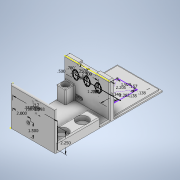
# Autodesk Inventor part: electropneumatic tray - rev2
Saved by Autodesk Inventor 2020 (Build 240168000, 168)
## iProperties
Created: 2022-01-12
Part Number: electropneumatic tray - rev2
Material: Generic
Document SubType Name: Modeling
Designer: pab2
Density: 1 g/cm^3
Appearance: Default
Author: pab2
Autodesk Inventor part; units mm, degrees
ref_plane "YZ Plane" through (0, 0, 0) normal (1, 0, 0) x (0, 1, 0)
ref_plane "XZ Plane" through (0, 0, 0) normal (0, 1, 0) x (-1, 0, 0)
ref_plane "XY Plane" through (0, 0, 0) normal (0, 0, 1) x (1, 0, 0)
sketch "Sketch1" plane through (0, 0, 0) normal (0, 0, 1) x (1, 0, 0)
  line L0 (0, 0) -> (127, 0)
  line L1 (127, 0) -> (127, 101.6)
  line L2 (127, 101.6) -> (0, 101.6)
  line L3 (0, 101.6) -> (0, 0)
  dimension "d0" = 127
  dimension "d1" = 101.6
  constraints: 8 end point, 2 parallel, 1 horizontal, 1 perpendicular
  measures "d0" distance of L2.end L1.end
  measures "d1" distance of L1.end L0.end
extrude "Extrusion1" add sketch "Sketch1" along normal blind 12.7
sketch "Sketch2" plane through (0, 0, 12.7) normal (0, 0, 1) x (1, 0, 0)
  line L0 (127, 101.6) -> (0, 101.6) projected
  line L1 (63.5, 101.6) -> (63.5, 69.85)
  line L2 (63.5, 69.85) -> (95.25, 69.85)
  line L3 (95.25, 69.85) -> (31.75, 69.85)
  circle A0 centre (31.75, 69.85) radius 9.906
  circle A1 centre (95.25, 69.85) radius 9.906
  line L4 (31.75, 63.5) -> (31.75, 76.2) construction
  line L5 (38.1, 63.5) -> (38.1, 76.2)
  line L6 (25.4, 76.2) -> (25.4, 63.5)
  arc A2 (25.4, 63.5) -> (38.1, 63.5) centre (31.75, 63.5) ccw
  arc A3 (38.1, 76.2) -> (25.4, 76.2) centre (31.75, 76.2) ccw
  line L7 (127, 69.85) -> (63.5, 69.85)
  circle A4 centre (63.5, 69.85) radius 9.906
  line L8 (69.85, 63.5) -> (69.85, 76.2)
  line L9 (57.15, 76.2) -> (57.15, 63.5)
  arc A5 (69.85, 76.2) -> (57.15, 76.2) centre (63.5, 76.2) ccw
  arc A6 (57.15, 63.5) -> (69.85, 63.5) centre (63.5, 63.5) ccw
  line L10 (158.75, 69.85) -> (95.25, 69.85)
  circle A7 centre (95.25, 69.85) radius 9.906
  line L11 (101.6, 63.5) -> (101.6, 76.2)
  line L12 (88.9, 76.2) -> (88.9, 63.5)
  arc A8 (101.6, 76.2) -> (88.9, 76.2) centre (95.25, 76.2) ccw
  arc A9 (88.9, 63.5) -> (101.6, 63.5) centre (95.25, 63.5) ccw
  point P0 (0, 0)
  point P1 (57.301, 62.1233)
  point P2 (69.699, 62.1233)
  point P3 (69.699, 77.5767)
  point P4 (57.301, 77.5767)
  dimension "d4" = 31.75
  dimension "d5" = 31.75
  dimension "d6" = 63.5
  dimension "d7" = 19.812
  dimension "d9" = 19.812
  dimension "d12" = 6.35
  dimension "d13" = 12.7
  dimension "d16" = 31.75
  constraints: 26 end point, 12 point on circle, 10 centre point, 4 coincident, 4 tangent, 2 midpoint, 2 perpendicular, 1 collinear, 1 horizontal, 1 parallel, 1 point on line, 1 vertical, 29 other
  measures "d4" distance of L1.start L1.end
  measures "d5" distance of L1.end L2.end
  measures "d6" distance of L2.end L3.end
  measures "d7" diameter of A0
  measures "d9" diameter of A1
  measures "d12" distance of A0.centre L4.end
  measures "d13" diameter of A3
  measures "d16" distance of L3.end L7.end
sketch "Sketch3" plane through (0, 0, 12.7) normal (0, 0, 1) x (1, 0, 0)
  line L0 (0, 101.6) -> (0, 0) projected
  line L1 (0, 0) -> (127, 0)
  line L2 (127, 0) -> (127, 6.35)
  line L3 (127, 6.35) -> (0, 6.35)
  line L4 (0, 6.35) -> (0, 0)
  dimension "d23" = 127
  dimension "d24" = 6.35
  constraints: 8 end point, 2 parallel, 1 horizontal, 1 perpendicular
  measures "d23" distance of L3.end L2.end
  measures "d24" distance of L2.end L1.end
extrude "Extrusion4" add sketch "Sketch3" along normal blind 152.4
sketch "Sketch4" plane through (0, 6.35, 12.7) normal (0, 1, 0) x (1, 0, 0)
  line L0 (127, 12.7) -> (127, -152.4) projected
  line L1 (0, 0) -> (0, -152.4) projected
  line L2 (127, -152.4) -> (0, -152.4)
  line L3 (0, -152.4) -> (0, -146.05)
  line L4 (0, -146.05) -> (127, -146.05)
  line L5 (127, -146.05) -> (127, -152.4)
  point P0 (0, 12.7)
  point P1 (0, -152.4)
  dimension "d27" = 6.35
  constraints: 8 end point, 2 parallel, 1 horizontal, 1 perpendicular, 1 point on line
  measures "d27" distance of L2.end L3.end
extrude "Extrusion5" add sketch "Sketch4" along normal blind 101.6
sketch "Sketch5" plane through (127, 6.35, 158.75) normal (0, 0, -1) x (-1, 0, 0)
  line L0 (127, 0) -> (127, 101.6) projected
  line L1 (127, 0) -> (0, 0)
  line L2 (0, 0) -> (0, 57.15)
  line L3 (0, 57.15) -> (127, 57.15)
  line L4 (127, 57.15) -> (127, 0)
  line L5 (63.5, 57.15) -> (63.5, 89.9922)
  line L6 (63.5, 57.15) -> (96.3422, 57.15) construction
  line L7 (63.5, 57.15) -> (72.5424, 57.15)
  line L8 (72.5424, 57.15) -> (72.5424, 65.6082)
  line L9 (72.5424, 65.6082) -> (54.4576, 65.6082)
  line L10 (127, 95.25) -> (127, -6.35) projected
  line L11 (127, -6.35) -> (76.2, -6.35)
  line L12 (76.2, -6.35) -> (76.2, 31.75)
  line L13 (76.2, 31.75) -> (127, 31.75)
  line L14 (127, 31.75) -> (127, -6.35)
  dimension "d30" = 127
  dimension "d31" = 57.15
  dimension "d32" = 32.8422
  dimension "d33" = 90
  dimension "d34" = 9.0424
  dimension "d35" = 8.4582
  dimension "d36" = 18.0848
  dimension "d120" = 50.8
  dimension "d121" = 38.1
  constraints: 26 end point, 5 perpendicular, 4 parallel, 3 horizontal, 1 coincident, 1 midpoint, 1 point on line, 1 vertical
  measures "d30" distance of L2.end L3.end
  measures "d31" distance of L1.end L2.end
  measures "d32" distance of L5.start L5.end
  measures "d33" angle of L6 L5
  measures "d34" distance of L5.start L7.end
  measures "d35" distance of L7.end L8.end
  measures "d36" distance of L8.end L9.end
  measures "d120" distance of L12.end L13.end
  measures "d121" distance of L11.end L12.end
hole "Hole1" at (63.5, 96.3422, 158.75) at (54.4576, 71.9582, 158.75) at (72.5424, 71.9582, 158.75) direction (0, 0, 1) diameter 3.4036 end through all clearance for "Socket Head Cap Screw" size "M3" standard "Ansi Metric M Profile"
sketch "Sketch10" plane through (0, 6.35, 12.7) normal (0, 1, 0) x (1, 0, 0)
  line L0 (127, 0) -> (127, -25.4)
  line L1 (127, 12.7) -> (127, -152.4) projected
  line L2 (127, -25.4) -> (88.9, -25.4)
  line L3 (88.9, -25.4) -> (88.9, -152.4)
  line L4 (88.9, -152.4) -> (127, -152.4)
  line L5 (127, -152.4) -> (127, -25.4)
  point P0 (0, 12.7)
  dimension "d58" = 25.4
  dimension "d59" = 38.1
  dimension "d60" = 127
  constraints: 10 end point, 2 parallel, 1 horizontal, 1 perpendicular, 1 point on line
  measures "d58" distance of L0.start L0.end
  measures "d59" distance of L4.end L3.end
  measures "d60" distance of L3.end L2.end
extrude "Extrusion9" add sketch "Sketch10" along normal blind 19.05
sketch "Sketch11" plane through (0, 25.4, 12.7) normal (0, 1, 0) x (1, 0, 0)
  line L0 (127, -25.4) -> (88.9, -25.4) projected
  line L1 (107.95, -25.4) -> (120.65, -25.4) construction
  circle A0 centre (107.95, -114.3) radius 16.51
  circle A1 centre (107.95, -57.15) radius 16.51
  line L2 (107.95, -25.4) -> (107.95, -57.15)
  line L3 (107.95, -25.4) -> (139.7, -25.4) construction
  line L4 (127, -146.05) -> (0, -146.05) projected
  line L5 (107.95, -146.05) -> (107.95, -114.3)
  line L6 (107.95, -146.05) -> (139.7, -146.05) construction
  point P0 (0, 12.7)
  dimension "d69" = 33.02
  dimension "d70" = 33.02
  dimension "d115" = 31.75
  dimension "d116" = 90
  dimension "d117" = 31.75
  dimension "d118" = 90
  constraints: 10 end point, 3 horizontal, 3 perpendicular, 2 centre point, 2 coincident, 1 midpoint, 1 point on line, 1 vertical
  measures "d69" diameter of A0
  measures "d70" diameter of A1
  measures "d115" distance of L1.start L2.end
  measures "d116" angle of L2 L3
  measures "d117" distance of L5.start L5.end
  measures "d118" angle of L6 L5
extrude "Extrusion10" cut sketch "Sketch11" against normal blind 12.7
sketch "Sketch12" plane through (0, 0, 0) normal (0, 0, -1) x (-1, 0, 0)
  line L0 (-127, 6.35) -> (-88.9, 6.35) projected
  line L1 (-127, 6.35) -> (0, 6.35)
  line L2 (0, 6.35) -> (0, 0)
  line L3 (0, 0) -> (-127, 0)
  line L4 (-127, 0) -> (-127, 6.35)
  constraints: 8 end point, 2 parallel, 1 horizontal, 1 perpendicular
extrude "Extrusion11" add sketch "Sketch12" along normal blind 137.16
sketch "Sketch13" plane through (0, 6.35, 0) normal (0, 1, 0) x (1, 0, 0)
  line L0 (35.5, 16.5925) -> (35.5, 101.5925)
  line L1 (35.5, 101.5925) -> (91.5, 101.5925)
  line L2 (91.5, 101.5925) -> (91.5, 16.5925)
  line L3 (91.5, 16.5925) -> (35.5, 16.5925)
  line L4 (35.5, 16.5925) -> (91.5, 101.5925) construction
  line L5 (35.5, 101.5925) -> (91.5, 16.5925) construction
  line L6 (91.5, 101.5925) -> (91.5, 98.0925)
  line L7 (91.5, 98.0925) -> (88, 98.0925)
  line L8 (88, 98.0925) -> (88, 101.5925)
  line L9 (88, 101.5925) -> (91.5, 101.5925)
  circle A0 centre (88, 98.0925) radius 2
  circle A1 centre (39, 98.0925) radius 2
  circle A2 centre (88, 40.0925) radius 2
  circle A3 centre (39, 40.0925) radius 2
  point P0 (0, 0)
  point P1 (63.5, 59.0925)
  dimension "d75" = 85
  dimension "d76" = 56
  dimension "d77" = 3.5
  dimension "d78" = 3.5
  dimension "d79" = 4
  dimension "d82" = 49
  dimension "d85" = 58
  constraints: 20 end point, 4 centre point, 4 coincident, 4 parallel, 2 midpoint, 2 perpendicular, 1 horizontal, 1 vertical, 9 other
  measures "d75" distance of L1.end L2.end
  measures "d76" distance of L0.end L1.end
  measures "d77" distance of L7.end L8.end
  measures "d78" distance of L6.end L7.end
  measures "d79" diameter of A0
  measures "d82" distance of A0.centre A1.centre
  measures "d85" distance of A0.centre A2.centre
extrude "Extrusion12" add sketch "Sketch13" along normal blind 3.175 contours A0 L7 L8 | L8 L7 A0 | A1 | A2 | A3
hole "Hole2" at (88, 6.35, -98.0925) at (39, 6.35, -98.0925) at (88, 6.35, -40.0925) at (39, 6.35, -40.0925) direction (0, 1, 0) diameter 2.013 depth 7.5946 tip angle 118 thread size "M2.5x0.45" class "6H" standard "ANSI Metric M Profile"
sketch "Sketch14" plane through (0, 6.35, 0) normal (0, 1, 0) x (1, 0, 0)
  line L0 (0, 137.16) -> (127, 137.16) projected
  line L1 (0, 0) -> (5.08, 0)
  line L2 (5.08, 0) -> (5.08, 137.16)
  line L3 (5.08, 137.16) -> (0, 137.16)
  line L4 (0, 137.16) -> (0, 0)
  line L5 (0, 137.16) -> (0, -165.1) projected
  line L6 (0, 137.16) -> (127, 137.16)
  line L7 (127, 137.16) -> (127, 132.08)
  line L8 (127, 132.08) -> (0, 132.08)
  line L9 (0, 132.08) -> (0, 137.16)
  line L10 (127, 137.16) -> (127, -165.1) projected
  line L11 (127, 0) -> (0, 0) projected
  line L12 (127, 137.16) -> (121.92, 137.16)
  line L13 (121.92, 137.16) -> (121.92, 0)
  line L14 (121.92, 0) -> (127, 0)
  line L15 (127, 0) -> (127, 137.16)
  point P0 (5.08, 132.08)
  point P1 (121.92, 132.08)
  dimension "d97" = 5.08
  dimension "d98" = 127
  dimension "d99" = 5.08
  dimension "d100" = 5.08
  constraints: 24 end point, 6 parallel, 3 horizontal, 3 perpendicular, 2 point on line
  measures "d97" distance of L3.end L2.end
  measures "d98" distance of L7.end L8.end
  measures "d99" distance of L6.end L7.end
  measures "d100" distance of L14.end L13.end
extrude "Extrusion13" cut sketch "Sketch14" against normal blind 3.175 contours L0 L2 L8 L4 | L0 L13 L8 L2 | L8 L2 L1 L4 | L0 L7 L8 L13 | L8 L10 L11 L13
sketch "Sketch15" plane through (0, 101.6, 0) normal (0, 1, 0) x (1, 0, 0)
  line L0 (121.92, 0) -> (5.08, 0) projected
  line L1 (63.5, 0) -> (63.5, -7.62)
  line L2 (88.9, -15.24) -> (38.1, -15.24)
  line L3 (38.1, -15.24) -> (38.1, 0)
  line L4 (38.1, 0) -> (88.9, 0)
  line L5 (88.9, 0) -> (88.9, -15.24)
  line L6 (88.9, -15.24) -> (38.1, 0) construction
  line L7 (38.1, -15.24) -> (88.9, 0) construction
  point P0 (0, 0)
  dimension "d103" = 7.62
  dimension "d104" = 50.8
  constraints: 14 end point, 3 midpoint, 2 parallel, 1 horizontal, 1 perpendicular, 1 point on line, 1 vertical
  measures "d103" distance of L1.start L1.end
  measures "d104" distance of L3.end L4.end
extrude "Extrusion14" cut sketch "Sketch15" against normal blind 5.08
sketch "Sketch16" plane through (0, 96.52, 0) normal (0, 1, 0) x (1, 0, 0)
  line L0 (38.1, -12.7) -> (38.1, 0) projected
  line L1 (38.1, 0) -> (63.5, 0)
  line L2 (121.92, 0) -> (5.08, 0) projected
  line L3 (63.5, 0) -> (63.5, -7.62)
  point P0 (0, 0)
  point P1 (38.1, -15.24)
  constraints: 4 end point, 1 midpoint, 1 vertical
hole "Hole3" at (63.5, 96.52, 7.62) direction (0, -1, 0) diameter 4.9784 depth 6.35 tip angle 118 thread size "1/4-20 UNC" class "2B" standard "ANSI Unified Screw Threads"
fillet "Fillet1" radius 3.175 11 edges at (0, 101.6, 6.35) (107.95, 101.6, 12.7) (19.05, 101.6, 12.7) (127, 101.6, 6.35) (127, 53.975, 12.7) (127, 6.35, 25.4) (0, 6.35, 85.725) (127, 66.675, 158.75) (63.5, 107.95, 158.75) (0, 57.15, 158.75) (63.5, 107.95, 165.1)
fillet "Fillet2" radius 3.175 7 edges at (127, 4.7628, 38.1) (127, 15.875, 38.1) (107.95, 25.4, 38.1) (127, 25.4, 98.425) (127, 25.4, 160.3372) (88.9, 25.4, 98.425) (88.9, 15.875, 38.1)
sketch "Sketch17" plane through (0, 0, 165.1) normal (0, 0, 1) x (1, 0, 0)
  point P0 (0, 0)
sketch "Sketch18" plane through (3.175, 6.35, 12.7) normal (0, 1, 0) x (1, 0, 0)
  line L0 (0, -146.05) -> (0, 0) projected
  line L1 (0, 0) -> (25.4, 0)
  line L2 (25.4, 0) -> (25.4, -25.4)
  line L3 (25.4, -25.4) -> (0, -25.4)
  line L4 (0, -25.4) -> (0, 0)
  point P0 (-3.175, 12.7)
  dimension "d129" = 25.4
  dimension "d130" = 25.4
  constraints: 8 end point, 2 parallel, 1 horizontal, 1 perpendicular
  measures "d129" distance of L2.end L3.end
  measures "d130" distance of L1.end L2.end
extrude "Extrusion15" add sketch "Sketch18" along normal blind 38.1
hole "Hole4" at (50.8, 38.1, 158.75) direction (0, 0, 1) diameter 8.89 end through all
sketch "Sketch19" plane through (3.175, 44.45, 12.7) normal (0, 1, 0) x (1, 0, 0)
  line L0 (25.4, -25.4) -> (0, -25.4) projected
  line L1 (0, -25.4) -> (12.7, -25.4)
  line L2 (12.7, -25.4) -> (12.7, -12.7)
  circle A0 centre (12.7, -12.7) radius 9.906
  point P0 (-3.175, 12.7)
  dimension "d133" = 12.7
  dimension "d134" = 12.7
  dimension "d135" = 90
  dimension "d136" = 19.812
  constraints: 4 end point, 1 centre point, 1 coincident, 1 midpoint, 1 perpendicular
  measures "d133" distance of L0.end L1.end
  measures "d134" distance of L1.end L2.end
  measures "d135" angle of L2 L1
  measures "d136" diameter of A0
extrude "Extrusion16" cut sketch "Sketch19" against normal blind 25.4
sketch "Sketch20" plane through (0, 0, 0) normal (0, 0, -1) x (-1, 0, 0)
  line L0 (-3.175, 44.45) -> (-28.575, 44.45) projected
  line L1 (-28.575, 44.45) -> (-28.575, 6.35) projected
  line L2 (-3.175, 6.35) -> (-3.175, 44.45) projected
  line L3 (-3.175, 6.35) -> (-3.175, 44.45) projected
  line L4 (-3.175, 44.45) -> (-28.575, 44.45) projected
  line L5 (-15.875, 44.45) -> (-15.875, 19.05)
  line L6 (-25.781, 19.05) -> (-5.969, 19.05) projected
  circle A0 centre (-15.875, 19.05) radius 3.175
  line L7 (-15.875, 19.05) -> (-41.275, 19.05)
  line L8 (-47.625, 19.05) -> (-34.925, 19.05) construction
  line L9 (-47.625, 15.875) -> (-34.925, 15.875)
  line L10 (-34.925, 22.225) -> (-47.625, 22.225)
  arc A1 (-47.625, 22.225) -> (-47.625, 15.875) centre (-47.625, 19.05) ccw
  arc A2 (-34.925, 15.875) -> (-34.925, 22.225) centre (-34.925, 19.05) ccw
  point P0 (0, 0)
  dimension "d139" = 25.4
  dimension "d140" = 6.35
  dimension "d143" = 25.4
  dimension "d144" = 6.35
  dimension "d145" = 6.35
  constraints: 12 end point, 4 point on circle, 4 tangent, 3 centre point, 3 midpoint, 2 point on line, 1 coincident, 1 parallel
  measures "d139" distance of L5.start L5.end
  measures "d140" diameter of A0
  measures "d143" distance of L7.start L7.end
  measures "d144" distance of L7.end L8.end
  measures "d145" diameter of A2
extrude "Extrusion17" cut sketch "Sketch20" against normal blind 31.75 contours A2 L9 A1 L10 | A0 L6 L5 | L5 L6 A0 | L6 A0
fillet "Fillet3" radius 1.5875 19 edges at (28.575, 25.4, 12.7) (28.575, 25.4, 38.1) (3.175, 25.4, 38.1) (15.875, 44.45, 38.1) (28.575, 44.45, 25.4) (3.175, 25.4, 12.7) (3.175, 44.45, 25.4) (0.9298, 100.6702, 11.7702) (0, 50.8005, 12.7) (50.8, 19.05, 12.7) (41.275, 15.875, 12.7) (31.75, 19.05, 12.7) (41.275, 22.225, 12.7) (31.75, 19.05, 0) (41.275, 15.875, 0) (50.8, 19.05, 0) (41.275, 22.225, 0) (19.05, 19.05, 0) (15.875, 44.45, 12.7)
body "Solid1"
